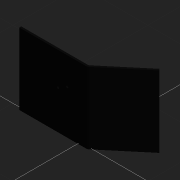
# Autodesk Inventor part: The Law Head
Saved by Autodesk Inventor 2015 SP1 (Build 190203100, 203)
## iProperties
Created: 2015-04-11
Part Number: The Law Head
Material: Aluminum 6061
Document SubType Name: Sheet Metal
Designer: datenney
Density: 2.7 g/cm^3
Sheet Metal Rule: Default
Appearance: Smooth - Black
Author: datenney
Autodesk Inventor part; units mm, degrees
ref_plane "YZ Plane" through (0, 0, 0) normal (1, 0, 0) x (0, 1, 0)
ref_plane "XZ Plane" through (0, 0, 0) normal (0, 1, 0) x (-1, 0, 0)
ref_plane "XY Plane" through (0, 0, 0) normal (0, 0, 1) x (1, 0, 0)
sketch "Sketch1" plane through (0, 0, 0) normal (0, 0, 1) x (1, 0, 0)
  line L0 (-88.9, -53.9686) -> (88.9, -53.9686)
  line L1 (88.9, -53.9686) -> (88.9, 53.9686)
  line L2 (88.9, 53.9686) -> (-88.9, 53.9686)
  line L3 (-88.9, 53.9686) -> (-88.9, -53.9686)
  line L4 (-88.9, -53.9686) -> (88.9, 53.9686) construction
  line L5 (88.9, -53.9686) -> (-88.9, 53.9686) construction
  line L6 (12.7, -53.9686) -> (12.7, 53.9686)
  point P0 (0, 0)
  dimension "d0" = 177.8
  dimension "d1" = 107.9373
  dimension "d2" = 76.2
  constraints: 14 end point, 2 midpoint, 2 parallel, 2 point on line, 1 horizontal, 1 perpendicular, 1 vertical
  measures "d0" distance of L2.end L1.end
  measures "d1" distance of L1.end L0.end
  measures "d2" distance between parallel lines of L1 L6
extrude "Plate1" add sketch "Sketch1" along normal blind 3.048
fold "Fold1" angle 40 bend radius 3.048 thickness 3.048 k factor 0.44 line from (12.7, -53.9686, 0) to (12.7, 53.9686, 0) line at bend centre moving side (1, 0, 0) folds toward (0, 0, -1)
sketch "Sketch2" plane through (0, 0, 0) normal (0, 0, -1) x (-1, 0, 0)
  circle A0 centre (218.6189, -101.5287) radius 2.4892 construction
  arc A1 (236.5187, -104.7811) -> (235.7654, -102.0548) centre (234.7789, -103.7946) ccw construction
  line L0 (235.7654, -102.0548) -> (15.5328, 22.8258) construction
  arc A2 (15.5328, 22.8258) -> (12.8065, 22.0725) centre (14.5462, 21.086) ccw projected
  line L1 (12.8065, 22.0725) -> (6.8874, 11.6339) projected
  arc A3 (6.8874, 11.6339) -> (7.6406, 8.9076) centre (8.6271, 10.6474) ccw projected
  line L2 (227.8733, -115.9729) -> (7.6406, 8.9076) construction
  arc A4 (227.8733, -115.9729) -> (230.5996, -115.2197) centre (228.8598, -114.2332) ccw construction
  line L3 (236.5187, -104.7811) -> (230.5996, -115.2197) construction
  circle A5 centre (225.5779, -105.4747) radius 1.85 construction
  circle A6 centre (211.6598, -97.5826) radius 1.85 construction
  circle A7 centre (197.7417, -89.6905) radius 1.85 construction
  circle A8 centre (183.8236, -81.7984) radius 1.85 construction
  circle A9 centre (169.9054, -73.9062) radius 1.85 construction
  circle A10 centre (155.9873, -66.0141) radius 1.85 construction
  circle A11 centre (142.0692, -58.122) radius 1.85 construction
  circle A12 centre (128.151, -50.2299) radius 1.85 construction
  circle A13 centre (114.2329, -42.3377) radius 1.85 construction
  circle A14 centre (100.3148, -34.4456) radius 1.85 construction
  circle A15 centre (86.3966, -26.5535) radius 1.85 projected
  circle A16 centre (72.4785, -18.6614) radius 1.85 projected
  circle A17 centre (58.5604, -10.7692) radius 1.85 projected
  circle A18 centre (44.6423, -2.8771) radius 1.85 projected
  circle A19 centre (30.7241, 5.015) radius 1.85 projected
  circle A20 centre (16.806, 12.9072) radius 1.85 projected
  line L4 (-11.1679, 53.9686) -> (-11.1679, -53.9686) projected
  line L5 (88.9, -53.9686) -> (-11.1679, -53.9686) projected
  line L6 (88.9, 53.9686) -> (88.9, -53.9686) projected
  line L7 (-11.1679, 53.9686) -> (88.9, 53.9686) projected
  line L8 (0, 0) -> (6.8874, 11.6339) construction
  line L9 (6.8874, 11.6339) -> (12.8065, 22.0725)
  line L10 (15.5328, 22.8258) -> (88.9, -18.7763)
  line L11 (88.9, -18.7763) -> (88.9, -37.1696)
  line L12 (88.9, -53.9686) -> (88.9, 53.9686) projected
  line L13 (88.9, -37.1696) -> (7.6406, 8.9076)
  arc A21 (6.8874, 11.6339) -> (7.6406, 8.9076) centre (8.6271, 10.6474) ccw
  arc A22 (15.5328, 22.8258) -> (12.8065, 22.0725) centre (14.5462, 21.086) ccw
  line L14 (88.9, -37.1696) -> (88.9, -53.9686)
  line L15 (88.9, -53.9686) -> (-11.1679, -53.9686)
  line L16 (-11.1679, -53.9686) -> (-11.1679, 53.9686)
  line L17 (-11.1679, 53.9686) -> (88.9, 53.9686)
  line L18 (88.9, 53.9686) -> (88.9, -53.9686)
  line L19 (-11.1679, 53.9686) -> (-70.3261, 53.9686)
  line L20 (-70.3261, 53.9686) -> (-70.3261, -53.9686)
  line L21 (-70.3261, -53.9686) -> (-11.1679, -53.9686)
  point P0 (13.793, 23.8123)
  dimension "d10" = 3.7
  dimension "d11" = 2
  constraints: 26 end point, 7 point on line, 6 tangent, 4 horizontal, 4 point on circle, 4 vertical, 2 centre point, 1 parallel
  measures "d10" diameter of A20
  measures "d11" radius of A22
hole "Hole1" at (70.3261, 53.9686, 0) at (70.3261, -53.9686, 0) at (-16.806, 12.9072, 0) at (-30.7241, 5.015, 0) direction (0, 0, 1) diameter 3.7084 end through all
equation "\"d1\" = 1.4165 * d2"
equation "\"d2\" = 0.428571 * d0"
equation "\"d4\" = BendReliefWidth"
equation "\"d5\" = BendReliefDepth"
equation "\"d6\" = MinimumRemnant"
equation "\"d7\" = BendRadius"
equation "\"d9\" = BendRadius"
equation "\"d17\" = Thickness"
equation "\"BendRadius\" = Thickness"
equation "\"BendReliefWidth\" = Thickness"
equation "\"BendReliefDepth\" = 0.5 * Thickness"
equation "\"CornerReliefSize\" = 4 * Thickness"
equation "\"MinimumRemnant\" = 2 * Thickness"
equation "\"TransitionRadius\" = BendRadius"
equation "\"JacobiRadiusSize\" = BendRadius"
equation "\"GapSize\" = Thickness"
equation "\"d3\" = BendRadius"
equation "\"Thickness\" = 3.048"
body "Solid1"
